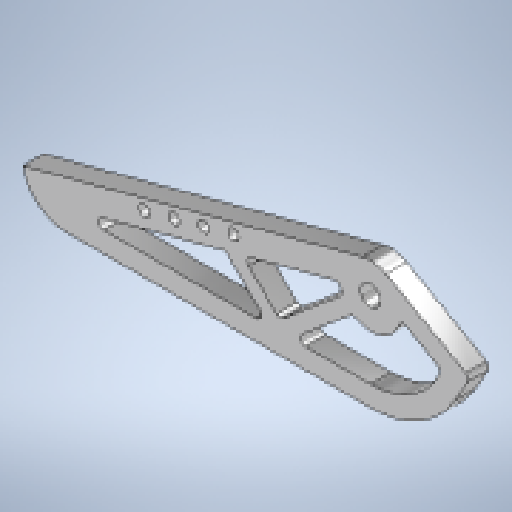
# Autodesk Inventor part: Arms
Saved by Autodesk Inventor 2023.2 (Build 272271000, 271)
## iProperties
Created: 2024-01-12
Part Number: Arms
Material: Aluminum 6061
Document SubType Name: Modeling
Designer: Nathan Cai
Mass: 26.2111 g
Surface Area: 51.1393 cm^2
Volume: 9.70782 cm^3
Density: 2.7 g/cm^3
Appearance: Aluminum - Flat
Author: Nathan Cai
Autodesk Inventor part; units mm, degrees
ref_plane "YZ Plane" through (0, 0, 0) normal (1, 0, 0) x (0, 1, 0)
ref_plane "XZ Plane" through (0, 0, 0) normal (0, 1, 0) x (-1, 0, 0)
ref_plane "XY Plane" through (0, 0, 0) normal (0, 0, 1) x (1, 0, 0)
sketch "Sketch2" plane through (0, 0, 0) normal (0, 0, 1) x (1, 0, 0)
  circle A0 centre (0, 0) radius 3.175
  circle A1 centre (0, 0) radius 6.35
  circle A2 centre (0, 0) radius 23.8125 construction
  line L0 (0, -23.8125) -> (0, 0) construction
  line L1 (0, 0) -> (20.6222, -11.9063) construction
  line L2 (20.6222, -11.9063) -> (4.5265, 4.4535)
  line L3 (-4.4901, 4.4901) -> (-24.8553, -15.875)
  line L4 (-24.8553, -15.875) -> (-88.9, -15.875)
  arc A3 (0, -23.8125) -> (20.6222, -11.9063) centre (0, 0) ccw
  line L5 (0, -23.8125) -> (-12.7, -23.8125)
  line L6 (-12.7, -23.8125) -> (-12.7, -30.1625)
  arc A4 (-88.9, -15.875) -> (-89.2282, -22.208) centre (-88.9, -19.05) ccw
  line L7 (-88.9, -19.05) -> (-88.9, -15.875) construction
  line L8 (-12.7, -30.1625) -> (-89.2282, -22.208)
  line L9 (-73.025, -15.875) -> (-46.0375, -15.875) construction
  line L10 (-46.0375, -15.875) -> (-46.0375, -20.6375) construction
  line L11 (-46.0375, -20.6375) -> (-73.025, -20.6375) construction
  line L12 (-73.025, -20.6375) -> (-73.025, -15.875) construction
  line L13 (-46.0375, -18.2563) -> (-73.025, -18.2563) construction
  circle A5 centre (-70.6437, -18.2563) radius 1.4732
  circle A6 centre (-64.2938, -18.2563) radius 1.4732
  circle A7 centre (-57.9438, -18.2563) radius 1.4732
  circle A8 centre (-51.5938, -18.2563) radius 1.4732
  circle A9 centre (-88.9, -19.05) radius 1.7526
  point P0 (-20.7184, -11.7381)
  dimension "d59" = 6.35
  dimension "d60" = 12.7
  dimension "d61" = 47.625
  dimension "d62" = 60
  dimension "d64" = 15.875
  dimension "d66" = 12.7
  dimension "d67" = 6.35
  dimension "d68" = 88.9
  dimension "d69" = 6.35
  dimension "d72" = 45
  dimension "d73" = 26.9875
  dimension "d74" = 4.7625
  dimension "d75" = 15.875
  dimension "d76" = 2.9464
  dimension "d77" = 2.3813
  dimension "d80" = 6.35
  dimension "d85" = 3.5052
  constraints: 29 end point, 10 centre point, 9 point on circle, 5 tangent, 4 coincident, 4 horizontal, 3 point on line, 2 concentric, 2 midpoint, 2 parallel, 2 vertical, 1 perpendicular, 6 other
  measures "d59" diameter of A0
  measures "d60" diameter of A1
  measures "d61" diameter of A2
  measures "d62" angle of L1 L0
  measures "d64" distance from line of L4 point (0, 0)
  measures "d66" distance from line of L0 L5.end
  measures "d67" distance of L5.end L6.end
  measures "d68" distance from line of L4.end L0
  measures "d69" diameter of A4
  measures "d72" angle of L0 L3
  measures "d73" distance of L10.end L11.end
  measures "d74" distance of L9.end L10.end
  measures "d75" distance between parallel lines of L7 L12
  measures "d76" diameter of A5
  measures "d77" distance from line of L12 A5.centre
  measures "d80" distance of A5.centre A6.centre
  measures "d85" diameter of A9
extrude "Extrusion2" add sketch "Sketch2" along normal blind 6.35
fillet "Fillet3" radius 12.7 1 edges at (-24.8553, -15.875, 3.175)
body "Solid2"
